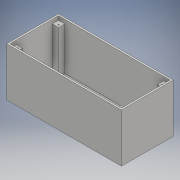
# Autodesk Inventor part: Box
Saved by Autodesk Inventor 2018.3 (Build 223285000, 285)
## iProperties
Created: 2022-01-12
Part Number: Box
Material: Generic
Document SubType Name: Modeling
Designer: Michael
Density: 1 g/cm^3
Appearance: Default
Author: Michael
Autodesk Inventor part; units mm, degrees
ref_plane "YZ Plane" through (0, 0, 0) normal (1, 0, 0) x (0, 1, 0)
ref_plane "XZ Plane" through (0, 0, 0) normal (0, 1, 0) x (-1, 0, 0)
ref_plane "XY Plane" through (0, 0, 0) normal (0, 0, 1) x (1, 0, 0)
sketch "Sketch1" plane through (0, 0, 0) normal (0, 0, 1) x (1, 0, 0)
  line L0 (-71, -31) -> (71, -31)
  line L1 (71, -31) -> (71, 31)
  line L2 (71, 31) -> (-71, 31)
  line L3 (-71, 31) -> (-71, -31)
  line L4 (-71, -31) -> (71, 31) construction
  line L5 (71, -31) -> (-71, 31) construction
  line L6 (-73, -33) -> (73, -33)
  line L7 (73, -33) -> (73, 33)
  line L8 (73, 33) -> (-73, 33)
  line L9 (-73, 33) -> (-73, -33)
  line L10 (-73, -33) -> (73, 33) construction
  line L11 (73, -33) -> (-73, 33) construction
  line L12 (-71, 31) -> (71, 31)
  line L13 (71, 31) -> (71, -31)
  line L14 (71, -31) -> (-71, -31)
  line L15 (-71, -31) -> (-71, 31)
  line L16 (-71, 31) -> (71, -31) construction
  line L17 (71, 31) -> (-71, -31) construction
  point P0 (0, 0)
  dimension "d0" = 142
  dimension "d1" = 62
  dimension "d2" = 2
  dimension "d3" = 2
  constraints: 36 end point, 6 midpoint, 6 parallel, 3 horizontal, 3 perpendicular
  measures "d0" distance of L2.end L1.end
  measures "d1" distance of L0.end L1.end
  measures "d2" distance between parallel lines of L2 L8
  measures "d3" distance between parallel lines of L7 L1
extrude "Extrusion1" add sketch "Sketch1" along normal blind 62
sketch "Sketch2" plane through (0, 0, 0) normal (0, 0, -1) x (-1, 0, 0)
  line L0 (71, -31) -> (-71, -31) projected
  line L1 (71, 31) -> (-71, 31)
  line L2 (-71, 31) -> (-71, -31)
  line L3 (-71, -31) -> (71, -31)
  line L4 (71, -31) -> (71, 31)
  line L5 (71, 31) -> (-71, -31) construction
  line L6 (-71, 31) -> (71, -31) construction
  point P0 (0, 0)
  constraints: 12 end point, 2 midpoint, 2 parallel, 1 horizontal, 1 perpendicular
extrude "Extrusion2" add sketch "Sketch2" against normal blind 2
sketch "Sketch3" plane through (0, 0, 2) normal (0, 0, 1) x (1, 0, 0)
  line L0 (-71, 31) -> (71, 31) projected
  line L1 (-71, 31) -> (-63, 31)
  line L2 (-63, 31) -> (-63, 23)
  line L3 (-63, 23) -> (-71, 23)
  line L4 (-71, 23) -> (-71, 31)
  line L5 (71, -31) -> (-71, -31) projected
  line L6 (-71, -31) -> (-63, -31)
  line L7 (-63, -31) -> (-63, -23)
  line L8 (-63, -23) -> (-71, -23)
  line L9 (-71, -23) -> (-71, -31)
  line L10 (71, 31) -> (71, -31) projected
  line L11 (71, 31) -> (63, 31)
  line L12 (63, 31) -> (63, 23)
  line L13 (63, 23) -> (71, 23)
  line L14 (71, 23) -> (71, 31)
  line L15 (71, 31) -> (71, -31) projected
  line L16 (71, -31) -> (63, -31)
  line L17 (63, -31) -> (63, -23)
  line L18 (63, -23) -> (71, -23)
  line L19 (71, -23) -> (71, -31)
  point P0 (0, 0)
  dimension "d8" = 8
  dimension "d9" = 8
  dimension "d10" = 8
  dimension "d11" = 8
  dimension "d12" = 8
  dimension "d13" = 8
  dimension "d14" = 8
  dimension "d15" = 8
  constraints: 32 end point, 8 parallel, 4 horizontal, 4 perpendicular
  measures "d8" distance of L2.end L3.end
  measures "d9" distance of L1.end L2.end
  measures "d10" distance of L8.end L7.end
  measures "d11" distance of L7.end L6.end
  measures "d12" distance of L13.end L12.end
  measures "d13" distance of L12.end L11.end
  measures "d14" distance of L17.end L18.end
  measures "d15" distance of L16.end L17.end
extrude "Extrusion3" add sketch "Sketch3" along normal blind 55
sketch "Sketch4" plane through (0, 0, 57) normal (0, 0, 1) x (1, 0, 0)
  circle A0 centre (-66, 26) radius 0.9
  circle A1 centre (66, 26) radius 0.9
  circle A2 centre (66, -26) radius 0.9
  circle A3 centre (-66, -26) radius 0.9
  line L0 (-71, 23) -> (-71, 31) projected
  line L1 (-71, 31) -> (-63, 31) projected
  line L2 (63, 31) -> (71, 31) projected
  line L3 (-71, -31) -> (-71, 31) projected
  point P0 (0, 0)
  dimension "d18" = 1.8
  dimension "d19" = 1.8
  dimension "d20" = 1.8
  dimension "d21" = 1.8
  dimension "d22" = 132
  dimension "d23" = 52
  dimension "d24" = 132
  dimension "d25" = 5
  dimension "d26" = 5
  dimension "d27" = 52
  dimension "d28" = 5
  dimension "d29" = 5
  constraints: 4 centre point
  measures "d18" diameter of A0
  measures "d19" diameter of A3
  measures "d20" diameter of A1
  measures "d21" diameter of A2
  measures "d22" distance of A1.centre A0.centre
  measures "d23" distance of A0.centre A3.centre
  measures "d24" distance of A3.centre A2.centre
  measures "d25" distance from line of L0 A0.centre
  measures "d26" distance from line of L1 A0.centre
  measures "d27" distance of A2.centre A1.centre
  measures "d28" distance from line of L2 A1.centre
  measures "d29" distance from line of L3 A3.centre
extrude "Extrusion4" cut sketch "Sketch4" against normal blind 20
equation "\"d10\" = d8"
equation "\"d11\" = d9"
equation "\"d12\" = d8"
equation "\"d13\" = d9"
equation "\"d14\" = d8"
equation "\"d15\" = d9"
equation "\"d19\" = d18"
equation "\"d20\" = d18"
equation "\"d21\" = d18"
equation "\"d24\" = d22"
equation "\"d25\" = d26"
equation "\"d27\" = d23"
equation "\"d28\" = d26"
equation "\"d29\" = d26"
body "Solid1"
